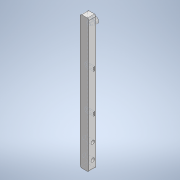
# Autodesk Inventor part: Arm
Saved by Autodesk Inventor 2021 (Build 250183000, 183)
## iProperties
Created: 2020-11-14
Part Number: Arm
Material: Generic
Document SubType Name: Modeling
Designer: siwat
Density: 1 g/cm^3
Appearance: Default
Author: siwat
Autodesk Inventor part; units mm, degrees
ref_plane "YZ Plane" through (0, 0, 0) normal (1, 0, 0) x (0, 1, 0)
ref_plane "XZ Plane" through (0, 0, 0) normal (0, 1, 0) x (-1, 0, 0)
ref_plane "XY Plane" through (0, 0, 0) normal (0, 0, 1) x (1, 0, 0)
sketch "Sketch1" plane through (0, 0, 0) normal (0, 0, 1) x (1, 0, 0)
  line L0 (-2.0384, 1.8879) -> (2.0592, 1.8879)
  line L1 (2.0592, 1.8879) -> (2.0592, -1.9739)
  line L2 (2.0592, -1.9739) -> (-2.0384, -1.9739)
  line L3 (-2.0384, -1.9739) -> (-2.0384, 1.8879)
  arc A0 (2.0592, -1.9739) -> (2.0592, 1.8879) centre (-0.1442, -0.043) ccw
  arc A1 (-2.0384, 1.8879) -> (-2.0384, -1.9739) centre (-0.6409, -0.043) ccw
  line L4 (6, 11.5957) -> (-6.1442, 11.5957)
  line L5 (-6.1442, 11.5957) -> (-6.1442, -176.351)
  line L6 (-6.1442, -176.351) -> (6, -176.351)
  line L7 (6, -176.351) -> (6, 11.5957)
  point P0 (0, 0)
  dimension "d2" = 6
  dimension "d3" = 6
  constraints: 16 end point, 4 parallel, 4 point on circle, 2 centre point, 2 horizontal, 2 perpendicular
  measures "d2" distance from line of L5 A0.centre
  measures "d3" distance from line of L7 point (0, 0)
extrude "Extrusion1" add sketch "Sketch1" along normal blind 10
sketch "Sketch2" plane through (-6.1442, -176.351, 0) normal (-1, 0, 0) x (0, 0, 1)
  line L0 (3.5426, 125.3505) -> (1.5426, 125.3505)
  line L1 (1.5426, 125.3505) -> (1.5426, 120.3505)
  line L2 (1.5426, 120.3505) -> (3.5426, 120.3505)
  line L3 (3.5426, 120.3505) -> (3.5426, 125.3505)
  line L4 (3.5426, 70.3505) -> (1.5426, 70.3505)
  line L5 (1.5426, 70.3505) -> (1.5426, 65.3505)
  line L6 (1.5426, 65.3505) -> (3.5426, 65.3505)
  line L7 (3.5426, 65.3505) -> (3.5426, 70.3505)
  circle A0 centre (4.5547, 34.075) radius 2.5
  circle A1 centre (4.5547, 12.3917) radius 2.5
  point P0 (0, 176.351)
  dimension "d4" = 2
  dimension "d5" = 5
  dimension "d6" = 2
  dimension "d7" = 5
  dimension "d10" = 50
  dimension "d11" = 5
  dimension "d12" = 5
  constraints: 16 end point, 4 parallel, 2 centre point, 2 horizontal, 2 perpendicular
  measures "d4" distance of L2.end L1.end
  measures "d5" distance of L2.end L0.start
  measures "d6" distance of L6.end L5.end
  measures "d7" distance of L6.end L4.start
  measures "d10" distance between parallel lines of L4 L2
  measures "d11" diameter of A0
  measures "d12" diameter of A1
extrude "Extrusion2" cut sketch "Sketch2" against normal through all
sketch "Sketch3" plane through (-6.1442, -176.351, 0) normal (-1, 0, 0) x (0, 0, 1)
  point P0 (0, 176.351)
sketch "Sketch4" plane through (0, 0, 0) normal (0, 0, -1) x (-1, 0, 0)
  circle A0 centre (0, 0) radius 4.5
  dimension "d13" = 9
  constraints: 1 centre point, 1 coincident
  measures "d13" diameter of A0
extrude "Extrusion3" add sketch "Sketch4" along normal blind 5.2375 and the other way blind 10
sketch "Sketch5" plane through (0, 0, 0) normal (0, 0, -1) x (-1, 0, 0)
  line L0 (2.0992, 1.8119) -> (-1.885, 1.8119)
  line L1 (-1.885, 1.8119) -> (-1.885, -1.9325)
  line L2 (-1.885, -1.9325) -> (2.0992, -1.9325)
  line L3 (2.0992, -1.9325) -> (2.0992, 1.8119)
  arc A0 (2.0992, -1.9325) -> (2.0992, 1.8119) centre (0.2308, -0.0603) ccw
  arc A1 (-1.885, 1.8119) -> (-1.885, -1.9325) centre (-0.0175, -0.0603) ccw
  point P0 (0, 0)
  constraints: 8 end point, 4 point on circle, 2 centre point, 2 parallel, 1 horizontal, 1 perpendicular
extrude "Extrusion4" cut sketch "Sketch5" along normal blind 5.2375 and the other way blind 4.2065
fillet "Fillet1" radius 2 4 edges at (6, 11.5957, 5) (-6.1442, 11.5957, 5) (-6.1442, -176.351, 5) (6, -176.351, 5)
body "Solid1"
